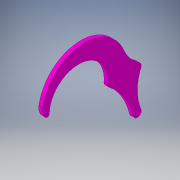
# Autodesk Inventor part: climb hook
Saved by Autodesk Inventor 2017 SP1 (Build 210196100, 196)
## iProperties
Created: 2018-03-18
Part Number: climb hook
Material: Aluminum 6061
Document SubType Name: Modeling
Designer: Ben
Density: 2.7 g/cm^3
Appearance: Magenta
Mass: 51.4695 g
Surface Area: 88.6391 cm^2
Volume: 19.0628 cm^3
Author: Ben
Autodesk Inventor part; units mm, degrees
ref_plane "YZ Plane" through (0, 0, 0) normal (1, 0, 0) x (0, 1, 0)
ref_plane "XZ Plane" through (0, 0, 0) normal (0, 1, 0) x (-1, 0, 0)
ref_plane "XY Plane" through (0, 0, 0) normal (0, 0, 1) x (1, 0, 0)
sketch "Sketch1" plane through (0, 0, 0) normal (1, 0, 0) x (0, 1, 0)
  line L0 (31.75, 0) -> (-31.75, 0) construction
  line L1 (-31.75, 0) -> (-31.75, -20.6375) construction
  line L2 (31.75, -20.6375) -> (31.75, 20.6375) construction
  circle A0 centre (31.75, -20.6375) radius 3.175
  circle A1 centre (31.75, 20.6375) radius 3.175
  circle A2 centre (-31.75, -20.6375) radius 3.175
  arc A3 (32.3103, 26.9627) -> (31.75, 121.7883) centre (36.5125, 74.402) ccw
  arc A4 (32.3103, 26.9627) -> (26.7051, 24.4939) centre (31.75, 20.6375) ccw
  arc A5 (-33.2262, -14.4615) -> (-29.3077, -26.499) centre (-31.75, -20.6375) ccw
  arc A6 (-33.2262, -14.4615) -> (26.7051, 24.4939) centre (-58.0173, 89.2573) ccw
  arc A7 (29.3077, -26.499) -> (37.057, -24.1244) centre (31.75, -20.6375) ccw
  arc A8 (29.3077, -26.499) -> (-29.3077, -26.499) centre (0, -96.8375) ccw
  line L3 (51.3987, 74.402) -> (36.5125, 74.402) construction
  arc A9 (52.0189, 132.2442) -> (31.75, 121.7883) centre (48.8804, 113.4545) ccw
  arc A10 (67.5698, 1.3552) -> (52.0189, 132.2442) centre (40.7089, 64.5321) ccw
  line L4 (48.8804, 113.4545) -> (50.8914, 119.8045) construction
  line L5 (67.5698, 1.3552) -> (55.1469, 30.5739) construction
  line L6 (-29.3077, -26.499) -> (-33.2262, -14.4615) construction
  line L7 (31.75, -20.6375) -> (-31.75, -20.6375) construction
  line L8 (25.9987, 99.802) -> (76.7987, 99.802)
  line L9 (76.7987, 99.802) -> (76.7987, 49.002)
  line L10 (76.7987, 49.002) -> (25.9987, 49.002)
  line L11 (25.9987, 49.002) -> (25.9987, 99.802)
  line L12 (25.9987, 99.802) -> (76.7987, 49.002) construction
  line L13 (76.7987, 99.802) -> (25.9987, 49.002) construction
  line L14 (48.8444, 120.4027) -> (52.0189, 132.2442) construction
  arc A11 (67.5698, 1.3552) -> (37.057, -24.1244) centre (94.4307, -61.8218) ccw
  point P0 (0, 0)
  point P1 (0, 0)
  point P2 (51.3987, 74.402)
  point P3 (51.3987, 74.402)
  dimension "d0" = 63.5
  dimension "d1" = 41.275
  dimension "d2" = 6.35
  dimension "d4" = 6.35
  dimension "d6" = 95.25
  dimension "d8" = 4.7625
  dimension "d9" = 19.05
  dimension "d10" = 6.35
  dimension "d12" = 31.75
  dimension "d21" = 50.8
  dimension "d24" = 0.508
  constraints: 30 end point, 22 point on circle, 12 centre point, 9 tangent, 7 coincident, 6 midpoint, 5 equal radius, 4 horizontal, 4 line through centre, 3 perpendicular, 2 parallel, 2 point on line, 1 vertical
  measures "d0" distance of L0.start L0.end
  measures "d1" distance of L2.start L2.end
  measures "d2" diameter of A0
  measures "d4" radius of A4
  measures "d6" diameter of A3
  measures "d8" distance from line of L2 L3.end
  measures "d9" radius of A9
  measures "d10" vertical distance of L4.start L4.end
  measures "d12" distance of L5.start L5.end
  measures "d21" distance of L10.end L8.start
  measures "d24" distance from line of L1.end L6
extrude "Extrusion1" add sketch "Sketch1" along normal blind 6.35 contours A3 A9 A10 A11 A7 A8 A5 A6 A4
fillet "Fillet2" radius 3.175 1 edges at (3.175, 31.75, 121.7883)
body "Solid1"
